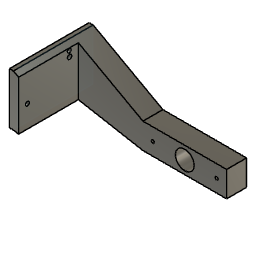
camera arm (Autodesk Fusion 360 design; units mm, degrees)
Autodesk Fusion 360 part; units mm, degrees
sketch "Sketch1" plane through (0, 0, 47.0945) normal (0, 0, 1) x (-1, 0, 0) in component "brat camera v5"
  arc A0 (-25.1826, -9.7) -> (-32.8174, -9.7) centre (-29, -14) ccw
  line L0 (-32.8174, -9.7) -> (-45.8466, -11.5241)
  arc A1 (-45.8466, -11.5241) -> (-45.8466, -16.4759) centre (-45.5, -14) ccw
  line L1 (-45.8466, -16.4759) -> (-32.8174, -18.3)
  arc A2 (-32.8174, -18.3) -> (-25.1826, -18.3) centre (-29, -14) ccw
  line L2 (-25.1826, -18.3) -> (-12.1534, -16.4759)
  arc A3 (-12.1534, -16.4759) -> (-12.1534, -11.5241) centre (-12.5, -14) ccw
  line L3 (-12.1534, -11.5241) -> (-25.1826, -9.7)
  circle A4 centre (-29, -14) radius 4.7
  circle A5 centre (-22, -14) radius 0.75
  circle A6 centre (-19, -14) radius 0.75
  circle A7 centre (-16, -14) radius 0.75
  circle A8 centre (-13, -14) radius 0.75
  circle A9 centre (-36, -14) radius 0.75
  circle A10 centre (-39, -14) radius 0.75
  circle A11 centre (-42, -14) radius 0.75
  circle A12 centre (-45, -14) radius 0.75
  circle A13 centre (-29, -14) radius 4.7
  circle A14 centre (-13, -14) radius 0.75
  circle A15 centre (-45, -14) radius 0.75
  line L4 (-8, -7.6137) -> (-50, -7.6137)
  line L5 (-50, -7.6137) -> (-50, -20.3863)
  line L6 (-50, -20.3863) -> (-8, -20.3863)
  line L7 (-8, -20.3863) -> (-8, -7.6137)
  line L8 (-8, -7.6137) -> (-50, -20.3863) construction
  line L9 (-50, -7.6137) -> (-8, -20.3863) construction
  line L10 (-8, -7.6137) -> (27, -7.6137)
  line L11 (27, -7.6137) -> (27, -20.3863)
  line L12 (27, -20.3863) -> (-8, -20.3863)
  line L13 (-8, -20.3863) -> (-8, -7.6137)
  line L14 (27, -7.6137) -> (27, 11.6736)
  line L15 (27, 11.6736) -> (-8, -7.6137)
  line L16 (-8, -20.3863) -> (27, -14)
  line L17 (24.4035, -20.3863) -> (24.4035, 10.2428)
  point P0 (-29, -14)
  dimension "d1_1" = 0
  dimension "d2" = 0
  dimension "d3" = 0
  dimension "d7" = 35
  constraint horizontal L4
  constraint perpendicular L4 L5
  constraint parallel L4 L6
  constraint parallel L5 L7
  constraint coincident L8 P0
  constraint coincident L9 P0
  constraint coincident P0 A0.centre
  constraint horizontal L10
  constraint vertical L11
  constraint horizontal L12
  constraint vertical L13
  constraint perpendicular L10 L14
  constraint midpoint L11 L16.end
  constraint coincident L12 L17.start
  constraint perpendicular L12 L17
  constraint coincident L15 L17.end
  measures "d7" distance of L4.start L10.end
sketch "Sketch2" plane through (0, 0, 47.0945) normal (0, 0, 1) x (-1, 0, 0) in component "brat camera v5"
sketch "Sketch3" plane through (0, 0, 47.0945) normal (0, 0, 1) x (-1, 0, 0) in component "brat camera v5"
sketch "Sketch4" plane through (0, 0, 47.0945) normal (0, 0, 1) x (-1, 0, 0) in component "brat camera v5"
sketch "Sketch5" plane through (0, 0, 47.0945) normal (0, 0, 1) x (-1, 0, 0) in component "brat camera v5"
sketch "Sketch6" plane through (0, 0, 47.0945) normal (0, 0, 1) x (-1, 0, 0) in component "brat camera v5"
sketch "Sketch7" plane through (0, 0, 47.0945) normal (0, 0, 1) x (1, 0, 0) in component "brat camera v5"
sketch "Sketch8" plane through (0, 0, 47.0945) normal (0, 0, 1) x (-1, 0, 0) in component "brat camera v5"
extrude "Extrude1" add sketch "Sketch1" against normal blind 25 contours L10 L14 L15 L17 | L10 L11 L16 L17 in component "brat camera v5"
extrude "Extrude2" add sketch "Sketch1" against normal blind 4 contours A0 L0 A1 L1 A2 L2 A3 L3 | A5 | A6 | A7 | A9 | A10 | A11 | L4 L5 L6 L7 L13 | L7 L10 L13 L16 L17 | L10 L15 L17 in component "brat camera v5"
extrude "Extrude3" add 1 faces at (-13.6024, 3.9482, 43.0945) along direction (0, 0, -1) blind 6 in component "brat camera v5"
extrude "Extrude4" add 1 faces at (-26.1345, -2.6388, 22.0945) along direction (0, 0, -1) blind 9 in component "brat camera v5"
extrude "Extrude5" add 1 faces at (-26.1345, -2.6388, 13.0945) along direction (0, 0, -1) blind 4 in component "brat camera v5"
sketch "Sketch9" plane through (-27, 0, 0) normal (-1, 0, 0) x (0, -1, 0) in component "brat camera v5"
  line L0 (11.6736, 47.0945) -> (-14, 47.0945)
  line L1 (-14, 47.0945) -> (-14, 9.0945)
  line L2 (-14, 9.0945) -> (11.6736, 9.0945)
  line L3 (11.6736, 9.0945) -> (11.6736, 47.0945)
sketch "Sketch10" plane through (-31.21, 0, 0) normal (-1, 0, 0) x (0, -1, 0) in component "brat camera v5"
  line L0 (-22.077, 33.9265) -> (-22.077, 12.1265)
  arc A0 (-22.077, 12.1265) -> (-20.477, 10.5265) centre (-20.477, 12.1265) ccw
  line L1 (-20.477, 10.5265) -> (-10.9709, 10.5265)
  arc A1 (-8.4092, 10.5265) -> (-10.9709, 10.5265) centre (-9.69, 12.5265) ccw
  line L2 (-8.4092, 10.5265) -> (-1.2959, 10.5265)
  arc A2 (1.785, 14.0759) -> (-1.2959, 10.5265) centre (-0.015, 12.5265) ccw
  line L3 (1.785, 14.0759) -> (1.785, 32.1771)
  arc A3 (-1.5644, 35.5265) -> (1.785, 32.1771) centre (-0.015, 33.7265) ccw
  line L4 (-1.5644, 35.5265) -> (-8.1407, 35.5265)
  arc A4 (-11.2394, 35.5265) -> (-8.1407, 35.5265) centre (-9.69, 33.7265) ccw
  line L5 (-11.2394, 35.5265) -> (-20.477, 35.5265)
  arc A5 (-20.477, 35.5265) -> (-22.077, 33.9265) centre (-20.477, 33.9265) ccw
  line L6 (-7.315, 17.6265) -> (-18.115, 17.6265)
  line L7 (-18.115, 17.6265) -> (-18.115, 28.4265)
  line L8 (-18.115, 28.4265) -> (-7.315, 28.4265)
  line L9 (-5.515, 29.5265) -> (-0.915, 29.5265)
  line L10 (-0.915, 29.5265) -> (-0.915, 20.5265)
  line L11 (-0.915, 20.5265) -> (-5.515, 20.5265)
  line L12 (-5.515, 20.5265) -> (-5.515, 29.5265)
sketch "Sketch11" plane through (-31.31, 0, 0) normal (-1, 0, 0) x (0, -1, 0) in component "brat camera v5"
  line L0 (-1.2959, 10.5265) -> (0.185, 10.5265)
  arc A0 (0.185, 10.5265) -> (1.785, 12.1265) centre (0.185, 12.1265) ccw
  line L1 (1.785, 12.1265) -> (1.785, 14.0759)
  arc A1 (1.785, 14.0759) -> (-1.2959, 10.5265) centre (-0.015, 12.5265) ccw
  circle A2 centre (-0.015, 12.5265) radius 1.1
  circle A3 centre (-0.015, 12.5265) radius 1.1
  dimension "d18" = 0
sketch "Sketch12" plane through (-31.31, 0, 0) normal (-1, 0, 0) x (0, -1, 0) in component "brat camera v5"
  arc A0 (-11.2394, 35.5265) -> (-8.1407, 35.5265) centre (-9.69, 33.7265) ccw
  line L0 (-8.1407, 35.5265) -> (-11.2394, 35.5265)
  circle A1 centre (-9.69, 33.7265) radius 1.1
  circle A2 centre (-9.69, 33.7265) radius 1.1
  dimension "d19" = 0
sketch "Sketch13" plane through (-31.31, 0, 0) normal (-1, 0, 0) x (0, -1, 0) in component "brat camera v5"
extrude "Extrude6" cut sketch "Sketch11" sketch "Sketch12" against normal blind 10 contours A2 A3 of sketch 2 contours A1 A2 in component "brat camera v5"
extrude "Extrude7" cut 1 faces at (-15.3333, 3.3134, 47.0945) along direction (0, 0, -1) blind 3 in component "brat camera v5"
extrude "Extrude8" cut sketch "Sketch9" against normal blind 3 in component "brat camera v5"
delete_face "DeleteFace1" 1 faces at (-26.1345, 14, 30.0945) in component "brat camera v5"
delete_face "DeleteFace2" 1 faces at (-13.3333, -4.1424, 39.4279) in component "brat camera v5"
extrude "Extrude9" add sketch "Sketch1" against normal blind 3 contours A0 L0 A1 L1 A2 L2 A3 L3 | A5 | A6 | A7 | A9 | A10 | A11 | L4 L5 L6 L7 L13 | L7 L10 L13 L16 L17 in component "brat camera v5"
extrude "Extrude10" cut 1 faces at (-24.4035, 12.1871, 45.0945) along direction (1, 0, 0) blind 0.4 in component "brat camera v5"
delete_face "DeleteFace3" 1 faces at (-2.6667, 18.44, 42.7612) in component "brat camera v5"
extrude "Extrude11" cut sketch "Sketch1" against normal blind 13 contours L7 L10 L13 L16 L17 | L12 L16 L17 in component "brat camera v5"
extrude "Extrude12" add sketch "Sketch1" against normal blind 10 contours L7 L10 L13 L16 L17 | L10 L15 L17 | L10 L14 L15 L17 | L10 L11 L16 L17 in component "brat camera v5"
extrude "Extrude13" cut sketch "Sketch1" against normal blind 37 contours L10 L14 L15 L17 | L10 L11 L16 L17 in component "brat camera v5"
extrude "Extrude14" add sketch "Sketch1" against normal blind 40 contours L10 L14 L15 L17 | L10 L11 L16 L17 in component "brat camera v5"
extrude "Extrude15" add 1 faces at (-27, 5.4421, 33.7612) along direction (-1, 0, 0) blind 2 in component "brat camera v5"
sketch "Sketch14" plane through (-29.3927, 0, 0) normal (-1, 0, 0) x (0, -1, 0) in component "brat camera v5"
  arc A0 (8.0307, 34.5) -> (11.0615, 31.4692) centre (9.0615, 32.5) ccw
  line L0 (11.0615, 31.4692) -> (11.0615, 32.5)
  arc A1 (11.0615, 32.5) -> (9.0615, 34.5) centre (9.0615, 32.5) ccw
  line L1 (9.0615, 34.5) -> (8.0307, 34.5)
  circle A2 centre (9.0615, 32.5) radius 1
  circle A3 centre (9.0615, 32.5) radius 1
  dimension "d41" = 0
sketch "Sketch15" plane through (-29.3927, 0, 0) normal (-1, 0, 0) x (0, -1, 0) in component "brat camera v5"
  arc A0 (-2.4077, 9.5) -> (-4.4693, 9.5) centre (-3.4385, 11.5) ccw
  line L0 (-4.4693, 9.5) -> (-2.4077, 9.5)
  circle A1 centre (-3.4385, 11.5) radius 1
  circle A2 centre (-3.4385, 11.5) radius 1
  dimension "d42" = 0
extrude "Extrude16" cut sketch "Sketch15" sketch "Sketch14" against normal blind 6 contours A1 A2 of sketch 2 contours A2 A3 in component "brat camera v5"
extrude "Extrude17" cut 1 faces at (-15.3333, 3.3134, 47.0945) along direction (0, 0, -1) blind 3 in component "brat camera v5"
extrude "Extrude18" add 1 faces at (-15.3333, 3.3134, 44.0945) along direction (0, 0, 1) blind 3 in component "brat camera v5"
sketch "sketch 2404" plane through (-35.9142, 41.37, 27.0748) normal (-1, 0, 0) x (0, 0, -1)
  line L0 (-4.08, 49.431) -> (-5.8294, 49.431)
  arc A0 (-5.8294, 49.431) -> (-7.4294, 47.831) centre (-5.8294, 47.831) ccw
  line L1 (-7.4294, 47.831) -> (-7.4294, 46.0816)
  arc A1 (-7.4294, 46.0816) -> (-4.08, 49.431) centre (-5.6294, 47.631) ccw
  circle A2 centre (-5.6294, 47.631) radius 1.1
  circle A3 centre (-5.6294, 47.631) radius 1.1
extrude "Extrude19" cut sketch "sketch 2404" against normal blind 15 contours A2 A3 in component "brat camera v5"
sketch "Sketch1 (2)" plane through (-35.9142, 0, 0) normal (-1, 0, 0) x (0, -1, 0)
  line L0 (-4.08, 49.431) -> (-5.8294, 49.431)
  arc A0 (-5.8294, 49.431) -> (-7.4294, 47.831) centre (-5.8294, 47.831) ccw
  line L1 (-7.4294, 47.831) -> (-7.4294, 46.0816)
  arc A1 (-7.4294, 46.0816) -> (-4.08, 49.431) centre (-5.6294, 47.631) ccw
  circle A2 centre (-5.6294, 47.631) radius 1.1
  circle A3 centre (-5.6294, 47.631) radius 1.1
  dimension "d1" = 0
component "brat camera v5" placed x (1, 0, 0) y (0, 0, -1) z (0, 1, 0) at (0, -27.0748, 41.37)
